Autodesk Fusion 360 part; units mm, degrees
(part 2 of 6)
  line L802 (34.113611, 287.460972) -> (34.113611, 286.790694)
  line L803 (27.199167, 285.555972) -> (27.128611, 285.59125)
  line L804 (18.485556, 226.85375) -> (18.626667, 226.783194)
  line L805 (12.311944, 223.114305) -> (12.206111, 223.149583)
  line L806 (40.675278, 262.907639) -> (40.675278, 263.260417)
  line L807 (41.557222, 261.672917) -> (41.310278, 261.708194)
  line L808 (41.310278, 261.708194) -> (41.169167, 261.814028)
  line L809 (25.011944, 250.454583) -> (25.047222, 250.384028)
  line L810 (35.277778, 273.490972) -> (34.713333, 275.325417)
  line L811 (34.713333, 275.325417) -> (34.148889, 273.490972)
  line L812 (34.148889, 273.490972) -> (35.277778, 273.490972)
  line L813 (31.75, 237.119583) -> (31.361944, 236.660972)
  line L814 (34.219444, 289.542361) -> (34.466389, 289.330694)
  line L815 (34.466389, 289.330694) -> (34.572222, 289.189583)
  line L816 (38.205833, 240.682639) -> (38.170556, 240.576805)
  line L817 (40.075556, 240.788472) -> (38.488056, 240.788472)
  line L818 (34.29, 287.990139) -> (34.395833, 287.990139)
  line L819 (39.123056, 244.457361) -> (39.017222, 244.457361)
  line L820 (25.964444, 250.419305) -> (25.999722, 250.384028)
  line L821 (25.964444, 253.312083) -> (25.964444, 250.595694)
  line L822 (32.243889, 286.190972) -> (32.490833, 285.90875)
  line L823 (32.490833, 285.90875) -> (32.808333, 285.697083)
  line L824 (24.659167, 285.59125) -> (24.553333, 285.626528)
  line L825 (31.361944, 231.969028) -> (31.4325, 231.93375)
  line L826 (41.310278, 264.777361) -> (41.557222, 264.847917)
  line L827 (41.169167, 261.814028) -> (40.922222, 262.166805)
  line L828 (40.922222, 262.166805) -> (40.781111, 262.590139)
  line L829 (38.770278, 244.210417) -> (38.735, 243.928194)
  line L830 (39.017222, 244.457361) -> (38.911389, 244.386805)
  line L831 (39.0525, 250.877917) -> (38.558611, 251.93625)
  line L832 (39.899167, 243.857639) -> (39.828611, 243.892917)
  line L833 (39.299444, 251.512917) -> (40.040278, 253.100417)
  line L834 (39.405278, 241.599861) -> (39.546389, 241.635139)
  line L835 (24.482778, 285.697083) -> (24.482778, 285.802917)
  line L836 (20.778611, 243.010972) -> (20.990278, 243.575417)
  line L837 (40.287222, 236.237639) -> (40.3225, 236.308194)
  line L838 (40.3225, 236.308194) -> (40.357778, 236.414028)
  line L839 (26.846389, 234.79125) -> (27.481389, 234.826528)
  line L840 (27.481389, 234.826528) -> (28.081111, 234.932361)
  line L841 (38.346944, 249.431528) -> (38.241111, 249.466805)
  line L842 (27.657778, 295.292639) -> (27.481389, 295.292639)
  line L843 (39.581667, 243.293194) -> (39.087778, 243.434305)
  line L844 (32.808333, 285.697083) -> (33.090556, 285.59125)
  line L845 (39.758056, 234.755972) -> (39.863889, 234.79125)
  line L846 (39.863889, 234.79125) -> (39.899167, 234.826528)
  line L847 (39.899167, 234.826528) -> (39.934444, 234.897083)
  line L848 (39.299444, 250.736805) -> (39.37, 250.772083)
  line L849 (39.37, 250.772083) -> (39.440556, 250.807361)
  line L850 (39.440556, 250.807361) -> (39.511111, 250.913194)
  line L851 (27.6225, 291.059305) -> (27.728333, 291.094583)
  line L852 (27.728333, 291.094583) -> (27.763611, 291.165139)
  line L853 (27.763611, 291.165139) -> (27.798889, 291.200417)
  line L854 (27.305, 291.200417) -> (27.340278, 291.129861)
  line L855 (39.934444, 234.897083) -> (39.934444, 235.002917)
  line L856 (38.664444, 234.755972) -> (39.652222, 234.755972)
  line L857 (22.577778, 229.252639) -> (22.507222, 229.429028)
  line L858 (22.507222, 229.429028) -> (22.507222, 229.605417)
  line L859 (34.113611, 238.107361) -> (34.360556, 238.742361)
  line L860 (28.081111, 247.385417) -> (27.481389, 247.455972)
  line L861 (27.481389, 247.455972) -> (26.846389, 247.49125)
  line L862 (40.005, 249.71375) -> (40.005, 249.607917)
  line L863 (40.005, 249.607917) -> (40.040278, 249.537361)
  line L864 (40.005, 251.93625) -> (40.005, 249.71375)
  line L865 (27.340278, 291.129861) -> (27.410833, 291.094583)
  line L866 (39.511111, 250.913194) -> (40.005, 251.93625)
  line L867 (29.845, 225.26625) -> (29.845, 223.643472)
  line L868 (16.051389, 286.825972) -> (16.051389, 286.296805)
  line L869 (27.516667, 228.723472) -> (27.410833, 228.723472)
  line L870 (20.990278, 243.575417) -> (21.2725, 244.139861)
  line L871 (39.0525, 226.85375) -> (38.170556, 226.85375)
  line L872 (34.113611, 293.634583) -> (34.007778, 293.52875)
  line L873 (28.716111, 247.244305) -> (29.280556, 247.032639)
  line L874 (20.990278, 238.707083) -> (20.778611, 239.306805)
  line L875 (41.874722, 261.77875) -> (41.945278, 261.884583)
  line L876 (34.713333, 241.494028) -> (34.713333, 240.788472)
  line L877 (34.713333, 240.788472) -> (34.678056, 240.118194)
  line L878 (34.678056, 240.118194) -> (34.536944, 239.412639)
  line L879 (34.536944, 239.412639) -> (34.360556, 238.742361)
  line L880 (34.360556, 238.742361) -> (34.113611, 238.107361)
  line L881 (34.113611, 238.107361) -> (33.831389, 237.472361)
  line L882 (33.831389, 237.472361) -> (33.478611, 236.872639)
  line L883 (33.478611, 236.872639) -> (33.055278, 236.308194)
  line L884 (33.055278, 236.308194) -> (32.596667, 235.779028)
  line L885 (32.596667, 235.779028) -> (32.102778, 235.285139)
  line L886 (32.102778, 235.285139) -> (31.573611, 234.861805)
  line L887 (31.573611, 234.861805) -> (31.009167, 234.438472)
  line L888 (31.009167, 234.438472) -> (30.374167, 234.120972)
  line L889 (30.374167, 234.120972) -> (29.739167, 233.83875)
  line L890 (29.739167, 233.83875) -> (29.104167, 233.591805)
  line L891 (29.104167, 233.591805) -> (28.398611, 233.450694)
  line L892 (28.398611, 233.450694) -> (27.728333, 233.344861)
  line L893 (27.728333, 233.344861) -> (27.022778, 233.274305)
  line L894 (27.022778, 233.274305) -> (26.317222, 233.309583)
  line L895 (26.317222, 233.309583) -> (25.646944, 233.380139)
  line L896 (25.646944, 233.380139) -> (24.976667, 233.52125)
  line L897 (24.976667, 233.52125) -> (24.306389, 233.697639)
  line L898 (24.306389, 233.697639) -> (23.636111, 233.979861)
  line L899 (23.636111, 233.979861) -> (23.036389, 234.262083)
  line L900 (23.036389, 234.262083) -> (22.436667, 234.650139)
  line L901 (22.436667, 234.650139) -> (21.872222, 235.073472)
  line L902 (21.872222, 235.073472) -> (21.343056, 235.532083)
  line L903 (21.343056, 235.532083) -> (20.884444, 236.025972)
  line L904 (20.884444, 236.025972) -> (20.461111, 236.590417)
  line L905 (20.461111, 236.590417) -> (20.073056, 237.154861)
  line L906 (20.073056, 237.154861) -> (19.755556, 237.789861)
  line L907 (19.755556, 237.789861) -> (19.473333, 238.424861)
  line L908 (19.473333, 238.424861) -> (19.261667, 239.095139)
  line L909 (19.261667, 239.095139) -> (19.120556, 239.765417)
  line L910 (19.120556, 239.765417) -> (19.014722, 240.470972)
  line L911 (19.014722, 240.470972) -> (18.979444, 241.14125)
  line L912 (18.979444, 241.14125) -> (19.014722, 241.846805)
  line L913 (19.014722, 241.846805) -> (19.120556, 242.552361)
  line L914 (19.120556, 242.552361) -> (19.261667, 243.222639)
  line L915 (19.261667, 243.222639) -> (19.473333, 243.892917)
  line L916 (19.473333, 243.892917) -> (19.755556, 244.527917)
  line L917 (19.755556, 244.527917) -> (20.073056, 245.127639)
  line L918 (20.073056, 245.127639) -> (20.461111, 245.727361)
  line L919 (20.461111, 245.727361) -> (20.884444, 246.291805)
  line L920 (20.884444, 246.291805) -> (21.343056, 246.785694)
  line L921 (21.343056, 246.785694) -> (21.872222, 247.244305)
  line L922 (21.872222, 247.244305) -> (22.436667, 247.667639)
  line L923 (22.436667, 247.667639) -> (23.036389, 248.020417)
  line L924 (23.036389, 248.020417) -> (23.636111, 248.337917)
  line L925 (23.636111, 248.337917) -> (24.306389, 248.584861)
  line L926 (24.306389, 248.584861) -> (24.976667, 248.796528)
  line L927 (24.976667, 248.796528) -> (25.646944, 248.937639)
  line L928 (25.646944, 248.937639) -> (26.317222, 249.008194)
  line L929 (26.317222, 249.008194) -> (27.022778, 249.043472)
  line L930 (27.022778, 249.043472) -> (27.728333, 248.972917)
  line L931 (27.728333, 248.972917) -> (28.398611, 248.867083)
  line L932 (28.398611, 248.867083) -> (29.104167, 248.690694)
  line L933 (29.104167, 248.690694) -> (29.739167, 248.479028)
  line L934 (29.739167, 248.479028) -> (30.374167, 248.196805)
  line L935 (30.374167, 248.196805) -> (31.009167, 247.844028)
  line L936 (31.009167, 247.844028) -> (31.573611, 247.455972)
  line L937 (31.573611, 247.455972) -> (32.102778, 247.032639)
  line L938 (32.102778, 247.032639) -> (32.596667, 246.53875)
  line L939 (32.596667, 246.53875) -> (33.055278, 246.009583)
  line L940 (33.055278, 246.009583) -> (33.478611, 245.445139)
  line L941 (33.478611, 245.445139) -> (33.831389, 244.845417)
  line L942 (33.831389, 244.845417) -> (34.113611, 244.210417)
  line L943 (34.113611, 244.210417) -> (34.360556, 243.540139)
  line L944 (34.360556, 243.540139) -> (34.536944, 242.869861)
  line L945 (34.536944, 242.869861) -> (34.678056, 242.199583)
  line L946 (34.678056, 242.199583) -> (34.713333, 241.494028)
  line L947 (1.446389, 282.945417) -> (14.322778, 295.821805)
  line L948 (39.828611, 243.963472) -> (39.793333, 244.034028)
  line L949 (15.980833, 223.643472) -> (16.086667, 223.537639)
  line L950 (39.934444, 243.822361) -> (39.899167, 243.857639)
  line L951 (39.087778, 243.434305) -> (39.581667, 243.293194)
  line L952 (33.161111, 240.541528) -> (33.090556, 239.906528)
  line L953 (39.793333, 244.034028) -> (39.6875, 244.31625)
  line L954 (29.280556, 247.032639) -> (28.716111, 247.244305)
  line L955 (28.716111, 247.244305) -> (28.081111, 247.385417)
  line L956 (40.216667, 243.892917) -> (40.146111, 243.822361)
  line L957 (39.0525, 265.624028) -> (39.123056, 265.694583)
  line L958 (33.408056, 289.824583) -> (32.949444, 289.71875)
  line L959 (32.949444, 289.71875) -> (32.596667, 289.542361)
  line L960 (20.672778, 295.821805) -> (19.261667, 295.821805)
  line L961 (13.899444, 289.048472) -> (6.596944, 281.745972)
  line L962 (43.285833, 281.745972) -> (43.991389, 282.486805)
  line L963 (25.153056, 229.675972) -> (25.576389, 231.087083)
  line L964 (40.251944, 243.963472) -> (40.216667, 243.892917)
  line L965 (15.5575, 225.372083) -> (15.522222, 225.336805)
  line L966 (27.446111, 285.732361) -> (27.410833, 285.661805)
  line L967 (23.459722, 289.824583) -> (21.2725, 289.824583)
  line L968 (37.076944, 261.602361) -> (37.076944, 261.567083)
  line L969 (27.163889, 289.471805) -> (27.093333, 289.365972)
  line L970 (30.1625, 295.11625) -> (30.091944, 295.186805)
  line L971 (30.091944, 295.186805) -> (30.021389, 295.257361)
  line L972 (30.021389, 295.257361) -> (29.809722, 295.292639)
  line L973 (26.387778, 252.077361) -> (26.387778, 253.20625)
  line L974 (23.918333, 251.265972) -> (24.341667, 252.677083)
  line L975 (24.765, 251.265972) -> (23.918333, 251.265972)
  line L976 (39.123056, 241.599861) -> (39.405278, 241.599861)
  line L977 (29.986111, 231.61625) -> (31.220833, 231.61625)
  line L978 (29.986111, 230.769583) -> (29.986111, 231.61625)
  line L979 (30.868056, 230.769583) -> (29.986111, 230.769583)
  line L980 (5.185833, 281.745972) -> (1.446389, 281.745972)
  line L981 (24.765, 289.648194) -> (24.729722, 289.577639)
  line L982 (25.294167, 289.612917) -> (25.153056, 289.754028)
  line L983 (36.5125, 226.959583) -> (36.477222, 227.030139)
  line L984 (37.853056, 289.71875) -> (37.958889, 289.789305)
  line L985 (30.338889, 250.525139) -> (30.338889, 253.382639)
  line L986 (30.127222, 250.313472) -> (30.233056, 250.313472)
  line L987 (27.305, 285.59125) -> (27.199167, 285.555972)
  line L988 (13.229167, 223.467083) -> (13.229167, 227.030139)
  line L989 (8.643056, 235.532083) -> (8.325556, 235.355694)
  line L990 (8.325556, 235.355694) -> (8.043333, 235.144028)
  line L991 (39.123056, 241.14125) -> (39.405278, 241.14125)
  line L992 (38.205833, 242.164305) -> (38.276389, 241.740972)
  line L993 (21.237222, 226.500972) -> (21.060833, 226.254028)
  line L994 (43.991389, 295.186805) -> (43.991389, 295.821805)
  line L995 (43.991389, 295.821805) -> (39.722778, 295.821805)
  line L996 (22.189722, 229.852361) -> (22.295556, 229.852361)
  line L997 (22.295556, 229.852361) -> (22.366111, 229.852361)
  line L998 (22.366111, 229.852361) -> (22.436667, 229.817083)
  line L999 (16.792222, 223.325972) -> (16.8275, 223.220139)
  line L1000 (16.8275, 223.220139) -> (16.898056, 223.149583)
  line L1001 (15.769167, 226.85375) -> (13.758333, 226.85375)
  line L1002 (38.311667, 228.794028) -> (38.4175, 228.75875)
  line L1003 (39.546389, 241.635139) -> (39.6875, 241.705694)
  line L1004 (15.804444, 227.382917) -> (13.581944, 227.382917)
  line L1005 (19.579167, 226.148194) -> (19.508611, 226.500972)
  line L1006 (19.508611, 226.500972) -> (19.332222, 226.85375)
  line L1007 (34.043056, 294.587083) -> (34.184167, 294.410694)
  line L1008 (9.913056, 223.467083) -> (9.913056, 223.36125)
  line L1009 (37.747222, 293.422917) -> (37.747222, 293.52875)
  line L1010 (37.747222, 293.52875) -> (37.711944, 293.599305)
  line L1011 (37.711944, 293.599305) -> (37.641389, 293.669861)
  line L1012 (16.051389, 226.924305) -> (16.086667, 226.994861)
  line L1013 (16.086667, 226.994861) -> (16.121944, 227.100694)
  line L1014 (22.154444, 229.217361) -> (22.083889, 229.570139)
  line L1015 (22.083889, 229.570139) -> (22.119167, 229.746528)
  line L1016 (22.119167, 229.746528) -> (22.189722, 229.852361)
  line L1017 (25.646944, 287.884305) -> (24.800278, 289.365972)
  line L1018 (27.763611, 291.165139) -> (27.728333, 291.094583)
  line L1019 (11.253611, 234.755972) -> (11.43, 234.403194)
  line L1020 (11.43, 234.403194) -> (11.535833, 234.085694)
  line L1021 (32.526111, 291.376805) -> (32.526111, 292.823194)
  line L1022 (13.335, 279.735139) -> (13.476111, 280.017361)
  line L1023 (39.6875, 244.31625) -> (39.793333, 244.034028)
  line L1024 (35.489444, 295.186805) -> (35.454167, 295.080972)
  line L1025 (35.665833, 226.889028) -> (35.418889, 226.85375)
  line L1026 (35.418889, 226.85375) -> (34.572222, 226.85375)
  line L1027 (29.950833, 294.79875) -> (29.809722, 294.763472)
  line L1028 (39.793333, 244.845417) -> (40.005, 244.669028)
  line L1029 (30.1625, 295.045694) -> (30.1625, 295.11625)
  line L1030 (39.934444, 243.822361) -> (40.040278, 243.787083)
  line L1031 (11.288889, 224.807639) -> (11.183056, 224.666528)
  line L1032 (3.104444, 222.549861) -> (1.446389, 220.891806)
  line L1033 (1.446389, 220.891806) -> (1.446389, 222.549861)
  line L1034 (1.446389, 222.549861) -> (3.104444, 222.549861)
  line L1035 (43.991389, 218.034306) -> (43.991389, 218.986806)
  line L1036 (8.043333, 235.144028) -> (7.796389, 234.897083)
  line L1037 (7.796389, 234.897083) -> (7.584722, 234.579583)
  line L1038 (7.584722, 234.579583) -> (7.443611, 234.262083)
  line L1039 (17.180278, 227.382917) -> (17.003889, 227.347639)
  line L1040 (17.003889, 227.347639) -> (16.862778, 227.277083)
  line L1041 (27.481389, 295.292639) -> (27.340278, 295.186805)
  line L1042 (27.340278, 295.186805) -> (27.305, 295.080972)
  line L1043 (27.305, 295.080972) -> (27.269722, 294.939861)
  line L1044 (29.809722, 295.292639) -> (27.657778, 295.292639)
  line L1045 (13.335, 257.898194) -> (13.229167, 258.180417)
  line L1046 (28.222222, 289.754028) -> (28.186944, 289.71875)
  line L1047 (28.398611, 248.867083) -> (27.728333, 248.972917)
  line L1048 (27.728333, 248.972917) -> (27.022778, 249.043472)
  line L1049 (27.022778, 249.043472) -> (26.317222, 249.008194)
  line L1050 (26.317222, 249.008194) -> (25.646944, 248.937639)
  line L1051 (36.5125, 227.277083) -> (36.477222, 227.241805)
  line L1052 (36.477222, 227.241805) -> (36.477222, 227.135972)
  line L1053 (39.0525, 227.382917) -> (36.83, 227.382917)
  line L1054 (34.219444, 292.999583) -> (34.572222, 293.352361)
  line L1055 (11.535833, 234.085694) -> (11.606389, 233.732917)
  line L1056 (8.748889, 223.396528) -> (8.748889, 223.255417)
  line L1057 (38.735, 244.810139) -> (39.087778, 244.915972)
  line L1058 (27.022778, 253.170972) -> (27.128611, 253.135694)
  line L1059 (8.043333, 235.144028) -> (8.325556, 235.355694)
  line L1060 (8.325556, 235.355694) -> (8.643056, 235.532083)
  line L1061 (35.595278, 272.432639) -> (35.630556, 272.362083)
  line L1062 (35.630556, 272.362083) -> (35.701111, 272.291528)
  line L1063 (39.087778, 244.915972) -> (39.405278, 244.95125)
  line L1064 (34.6075, 289.08375) -> (34.572222, 289.189583)
  line L1065 (34.572222, 289.189583) -> (34.466389, 289.330694)
  line L1066 (34.078333, 285.732361) -> (34.29, 285.90875)
  line L1067 (34.29, 285.90875) -> (34.466389, 286.085139)
  line L1068 (31.220833, 229.111528) -> (29.986111, 229.111528)
  line L1069 (31.467778, 228.899861) -> (31.467778, 228.970417)
  line L1070 (31.467778, 228.970417) -> (31.4325, 229.040972)
  line L1071 (38.523333, 253.135694) -> (38.452778, 253.170972)
  line L1072 (38.452778, 253.170972) -> (38.4175, 253.20625)
  line L1073 (38.4175, 253.20625) -> (38.346944, 253.20625)
  line L1074 (25.964444, 288.44875) -> (26.67, 289.648194)
  line L1075 (27.6225, 231.61625) -> (27.6225, 230.769583)
  line L1076 (37.288611, 261.14375) -> (37.359167, 261.14375)
  line L1077 (7.443611, 234.262083) -> (7.337778, 233.909305)
  line L1078 (7.337778, 233.909305) -> (7.3025, 233.52125)
  line L1079 (36.935833, 281.745972) -> (31.996944, 281.745972)
  line L1080 (12.453056, 223.149583) -> (12.311944, 223.114305)
  line L1081 (19.085278, 223.290694) -> (19.191111, 223.184861)
  line L1082 (19.191111, 223.184861) -> (19.296944, 223.149583)
  line L1083 (40.146111, 243.822361) -> (40.216667, 243.892917)
  line L1084 (16.862778, 227.277083) -> (16.792222, 227.135972)
  line L1085 (15.5575, 225.58375) -> (15.5575, 225.513194)
  line L1086 (30.374167, 248.196805) -> (29.739167, 248.479028)
  line L1087 (29.739167, 248.479028) -> (29.104167, 248.690694)
  line L1088 (29.104167, 248.690694) -> (28.398611, 248.867083)
  line L1089 (27.375556, 286.014583) -> (26.281944, 287.884305)
  line L1090 (27.446111, 285.802917) -> (27.446111, 285.944028)
  line L1091 (27.375556, 284.885694) -> (24.235833, 281.745972)
  line L1092 (13.440833, 223.114305) -> (13.581944, 223.114305)
  line L1093 (13.229167, 227.030139) -> (13.229167, 223.467083)
  line L1094 (13.581944, 227.382917) -> (13.440833, 227.347639)
  line L1095 (38.488056, 249.502083) -> (38.4175, 249.466805)
  line L1096 (15.804444, 223.643472) -> (15.875, 223.643472)
  line L1097 (22.824722, 236.237639) -> (22.366111, 236.660972)
  line L1098 (40.357778, 242.234861) -> (40.287222, 242.622917)
  line L1099 (40.287222, 242.622917) -> (40.110833, 242.975694)
  line L1100 (40.110833, 242.975694) -> (39.899167, 243.187361)
  line L1101 (39.899167, 243.187361) -> (39.581667, 243.293194)
  line L1102 (34.642778, 265.200694) -> (33.584444, 261.567083)
  line L1103 (34.925, 265.377083) -> (34.819167, 265.377083)
  line L1104 (38.523333, 242.481805) -> (38.593889, 242.41125)
  line L1105 (23.530278, 229.358472) -> (23.389167, 229.182083)
  line L1106 (23.424444, 230.064028) -> (23.530278, 229.852361)
  line L1107 (33.584444, 272.25625) -> (33.690278, 272.25625)
  line L1108 (33.690278, 272.25625) -> (33.760833, 272.291528)
  line L1109 (21.872222, 235.073472) -> (22.436667, 234.650139)
  line L1110 (22.436667, 234.650139) -> (23.036389, 234.262083)
  line L1111 (23.036389, 234.262083) -> (23.636111, 233.979861)
  line L1112 (1.446389, 219.445417) -> (4.550833, 222.549861)
  line L1113 (4.550833, 222.549861) -> (9.454444, 222.549861)
  line L1114 (36.583056, 226.889028) -> (36.5125, 226.959583)
  line L1115 (38.523333, 249.537361) -> (38.558611, 249.749028)
  line L1116 (38.1, 249.749028) -> (38.135278, 249.537361)
  line L1117 (38.135278, 249.537361) -> (38.170556, 249.502083)
  line L1118 (38.170556, 249.502083) -> (38.241111, 249.466805)
  line L1119 (31.996944, 291.412083) -> (31.996944, 291.30625)
  line L1120 (34.007778, 272.961805) -> (35.418889, 272.961805)
  line L1121 (33.831389, 272.397361) -> (34.007778, 272.961805)
  line L1122 (33.655, 293.352361) -> (33.443333, 293.352361)
  line L1123 (25.999722, 250.384028) -> (26.070278, 250.313472)
  line L1124 (26.070278, 250.313472) -> (26.176111, 250.313472)
  line L1125 (15.522222, 225.336805) -> (15.451667, 225.301528)
  line L1126 (38.346944, 253.20625) -> (38.4175, 253.20625)
  line L1127 (38.276389, 240.753194) -> (38.488056, 240.788472)
  line L1128 (39.017222, 237.190139) -> (39.017222, 237.33125)
  line L1129 (27.798889, 291.200417) -> (27.763611, 291.165139)
  line L1130 (30.338889, 253.382639) -> (30.303611, 253.488472)
  line L1131 (30.303611, 253.488472) -> (30.268333, 253.559028)
  line L1132 (37.359167, 261.14375) -> (37.429722, 261.179028)
  line L1133 (37.429722, 261.179028) -> (37.500278, 261.284861)
  line L1134 (27.128611, 252.147917) -> (27.022778, 252.112639)
  line L1135 (27.022778, 252.112639) -> (26.881667, 252.077361)
  line L1136 (26.881667, 252.077361) -> (26.387778, 252.077361)
  line L1137 (26.916944, 253.20625) -> (27.022778, 253.170972)
  line L1138 (30.303611, 250.454583) -> (30.338889, 250.525139)
  line L1139 (29.950833, 250.384028) -> (29.986111, 250.34875)
  line L1140 (39.0525, 230.310972) -> (39.899167, 228.864583)
  line L1141 (21.237222, 226.500972) -> (21.448889, 226.712639)
  line L1142 (21.448889, 226.712639) -> (21.695833, 226.818472)
  line L1143 (21.695833, 226.818472) -> (21.9075, 226.85375)
  line L1144 (28.469167, 253.594305) -> (28.539722, 253.594305)
  line L1145 (25.999722, 253.52375) -> (25.964444, 253.417917)
  line L1146 (25.964444, 253.417917) -> (25.964444, 253.312083)
  line L1147 (30.056667, 253.594305) -> (30.021389, 253.559028)
  line L1148 (30.021389, 253.559028) -> (29.950833, 253.488472)
  line L1149 (27.199167, 252.183194) -> (27.128611, 252.147917)
  line L1150 (20.496389, 241.14125) -> (20.531667, 241.77625)
  line L1151 (31.009167, 234.438472) -> (31.573611, 234.861805)
  line L1152 (31.573611, 234.861805) -> (32.102778, 235.285139)
  line L1153 (32.102778, 235.285139) -> (32.596667, 235.779028)
  line L1154 (31.361944, 245.656805) -> (31.75, 245.198194)
  line L1155 (27.798889, 291.376805) -> (27.798889, 291.30625)
  line L1156 (26.846389, 234.79125) -> (26.246667, 234.826528)
  line L1157 (33.655, 287.990139) -> (34.29, 287.990139)
  line L1158 (30.233056, 250.313472) -> (30.303611, 250.384028)
  line L1159 (30.303611, 250.384028) -> (30.303611, 250.454583)
  line L1160 (38.276389, 240.365139) -> (38.452778, 240.329861)
  line L1161 (38.488056, 240.788472) -> (38.276389, 240.753194)
  line L1162 (38.276389, 240.753194) -> (38.241111, 240.717917)
  line L1163 (38.241111, 240.717917) -> (38.205833, 240.682639)
  line L1164 (31.996944, 294.939861) -> (31.996944, 291.412083)
  line L1165 (32.385, 295.292639) -> (32.208611, 295.292639)
  line L1166 (16.051389, 286.296805) -> (11.535833, 281.745972)
  line L1167 (39.0525, 237.154861) -> (39.017222, 237.190139)
  line L1168 (39.616944, 244.915972) -> (39.440556, 244.95125)
  line L1169 (40.287222, 244.034028) -> (40.216667, 244.280972)
  line L1170 (40.216667, 244.280972) -> (40.146111, 244.457361)
  line L1171 (40.040278, 243.787083) -> (40.146111, 243.822361)
  line L1172 (22.789444, 229.111528) -> (22.718889, 229.146805)
  line L1173 (22.718889, 229.146805) -> (22.577778, 229.252639)
  line L1174 (34.6075, 286.367361) -> (34.642778, 286.614305)
  line L1175 (35.348333, 285.873472) -> (35.348333, 285.732361)
  line L1176 (35.348333, 285.732361) -> (35.418889, 285.626528)
  line L1177 (35.418889, 285.626528) -> (35.489444, 285.59125)
  line L1178 (16.792222, 227.135972) -> (16.792222, 226.994861)
  line L1179 (18.273889, 227.382917) -> (17.180278, 227.382917)
  line L1180 (21.343056, 235.532083) -> (21.872222, 235.073472)
  line L1181 (31.115, 230.628472) -> (31.079722, 230.699028)
  line L1182 (31.079722, 230.699028) -> (31.044444, 230.734305)
  line L1183 (31.044444, 230.734305) -> (30.868056, 230.769583)
  line L1184 (38.205833, 240.682639) -> (38.241111, 240.717917)
  line L1185 (32.138056, 237.613472) -> (32.455556, 238.177917)
  line L1186 (32.455556, 238.177917) -> (32.737778, 238.707083)
  line L1187 (4.974167, 218.034306) -> (1.446389, 218.034306)
  line L1188 (1.446389, 218.034306) -> (1.446389, 219.445417)
  line L1189 (39.722778, 295.821805) -> (39.334722, 295.43375)
  line L1190 (39.334722, 290.494861) -> (43.991389, 295.186805)
  line L1191 (27.587222, 223.749305) -> (27.834167, 223.925694)
  line L1192 (27.375556, 223.67875) -> (27.587222, 223.749305)
  line L1193 (21.448889, 287.707917) -> (21.448889, 286.085139)
  line L1194 (21.448889, 286.085139) -> (23.495, 286.085139)
  line L1195 (23.495, 286.085139) -> (23.565556, 286.085139)
  line L1196 (33.760833, 292.823194) -> (34.219444, 292.999583)
  line L1197 (12.135556, 223.184861) -> (12.065, 223.255417)
  line L1198 (37.923611, 222.549861) -> (41.204444, 222.549861)
  line L1199 (42.650833, 222.549861) -> (43.991389, 222.549861)
  line L1200 (43.991389, 222.549861) -> (43.991389, 281.745972)
  line L1201 (39.228889, 265.694583) -> (39.299444, 265.659305)
  line L1202 (29.986111, 250.34875) -> (30.021389, 250.313472)
  line L1203 (30.021389, 250.313472) -> (30.127222, 250.313472)
  line L1204 (34.854444, 222.549861) -> (30.374167, 218.034306)
  line L1205 (30.374167, 218.034306) -> (25.435278, 218.034306)
  line L1206 (25.435278, 218.034306) -> (29.950833, 222.549861)
  line L1207 (29.950833, 222.549861) -> (31.855833, 222.549861)
  line L1208 (33.760833, 272.291528) -> (33.796111, 272.326805)
  line L1209 (33.796111, 272.326805) -> (33.831389, 272.397361)
  line L1210 (33.302222, 272.467917) -> (33.3375, 272.362083)
  line L1211 (38.241111, 291.094583) -> (37.958889, 291.059305)
  line L1212 (35.348333, 289.577639) -> (35.348333, 289.507083)
  line L1213 (35.56, 289.824583) -> (35.489444, 289.789305)
  line L1214 (35.489444, 289.789305) -> (35.418889, 289.754028)
  line L1215 (20.6375, 239.906528) -> (20.778611, 239.306805)
  line L1216 (20.778611, 239.306805) -> (20.990278, 238.707083)
  line L1217 (29.315833, 285.732361) -> (29.315833, 285.838194)
  line L1218 (24.765, 289.648194) -> (24.800278, 289.71875)
  line L1219 (16.121944, 223.255417) -> (16.157222, 223.396528)
  line L1220 (13.581944, 223.114305) -> (15.769167, 223.114305)
  line L1221 (13.229167, 223.467083) -> (13.264444, 223.325972)
  line L1222 (39.0525, 265.624028) -> (38.981944, 265.553472)
  line L1223 (42.051111, 262.343194) -> (42.015833, 262.131528)
  line L1224 (17.885833, 224.913472) -> (19.085278, 223.290694)
  line L1225 (17.321389, 224.913472) -> (17.885833, 224.913472)
  line L1226 (17.321389, 223.467083) -> (17.321389, 224.913472)
  line L1227 (17.074444, 223.114305) -> (17.180278, 223.149583)
  line L1228 (29.845, 225.760139) -> (31.326667, 225.760139)
  line L1229 (24.800278, 289.71875) -> (24.906111, 289.789305)
  line L1230 (13.758333, 225.26625) -> (13.758333, 223.643472)
  line L1231 (31.397222, 228.75875) -> (31.4325, 228.75875)
  line L1232 (17.180278, 223.149583) -> (17.215556, 223.184861)
  line L1233 (17.215556, 223.184861) -> (17.286111, 223.220139)
  line L1234 (39.264167, 237.01375) -> (39.334722, 237.01375)
  line L1235 (39.334722, 237.01375) -> (39.405278, 237.049028)
  line L1236 (39.405278, 237.049028) -> (39.475833, 237.119583)
  line L1237 (39.475833, 237.119583) -> (39.511111, 237.295972)
  line L1238 (9.383889, 235.673194) -> (8.995833, 235.637917)
  line L1239 (8.995833, 235.637917) -> (8.643056, 235.532083)
  line L1240 (12.065, 223.255417) -> (12.065, 223.325972)
  line L1241 (22.507222, 223.960972) -> (22.577778, 224.137361)
  line L1242 (29.5275, 293.246528) -> (29.421667, 293.21125)
  line L1243 (34.360556, 288.695694) -> (34.501667, 288.730972)
  line L1244 (34.501667, 288.730972) -> (34.572222, 288.801528)
  line L1245 (28.2575, 253.347361) -> (28.292778, 253.488472)
  line L1246 (37.429722, 293.705139) -> (37.641389, 293.669861)
  line L1247 (31.4325, 228.75875) -> (31.467778, 228.829305)
  line L1248 (31.467778, 228.829305) -> (31.467778, 228.899861)
  line L1249 (29.845, 228.723472) -> (31.220833, 228.723472)
  line L1250 (38.523333, 236.660972) -> (40.075556, 236.660972)
  line L1251 (24.906111, 289.789305) -> (25.011944, 289.824583)
  line L1252 (12.065, 223.325972) -> (12.065, 223.431805)
  line L1253 (13.264444, 223.325972) -> (13.335, 223.184861)
  line L1254 (13.335, 223.184861) -> (13.440833, 223.114305)
  line L1255 (35.454167, 294.939861) -> (35.454167, 291.376805)
  line L1256 (32.243889, 258.497917) -> (32.208611, 258.180417)
  line L1257 (35.418889, 289.754028) -> (35.348333, 289.648194)
  line L1258 (37.958889, 294.763472) -> (38.1, 294.763472)
  line L1259 (38.1, 294.763472) -> (38.205833, 294.834028)
  line L1260 (11.43, 234.403194) -> (11.253611, 234.755972)
  line L1261 (11.253611, 234.755972) -> (11.006667, 235.038194)
  line L1262 (38.276389, 294.869305) -> (38.205833, 294.834028)
  line L1263 (29.598056, 228.970417) -> (29.598056, 228.864583)
  line L1264 (29.598056, 228.864583) -> (29.668611, 228.75875)
  line L1265 (29.668611, 228.75875) -> (29.739167, 228.723472)
  line L1266 (39.581667, 230.310972) -> (39.616944, 230.34625)
  line L1267 (40.216667, 229.182083) -> (39.581667, 230.310972)
  line L1268 (40.251944, 229.146805) -> (40.216667, 229.182083)
  line L1269 (40.3225, 228.970417) -> (40.3225, 229.040972)
  line L1270 (40.3225, 229.040972) -> (40.287222, 229.07625)
  line L1271 (30.021389, 295.257361) -> (30.091944, 295.186805)
  line L1272 (38.170556, 249.502083) -> (38.135278, 249.537361)
  line L1273 (27.269722, 291.376805) -> (27.269722, 294.939861)
  line L1274 (25.047222, 250.384028) -> (25.117778, 250.313472)
  line L1275 (21.59, 237.613472) -> (21.2725, 238.177917)
  line L1276 (32.243889, 279.135417) -> (32.243889, 258.497917)
  line L1277 (19.120556, 242.552361) -> (19.014722, 241.846805)
  line L1278 (19.014722, 241.846805) -> (18.979444, 241.14125)
  line L1279 (23.565556, 230.487361) -> (23.318611, 230.593194)
  line L1280 (23.142222, 228.723472) -> (23.530278, 228.794028)
  line L1281 (23.671389, 247.526528) -> (23.106944, 247.209028)
  line L1282 (23.106944, 247.209028) -> (22.577778, 246.820972)
  line L1283 (20.990278, 243.575417) -> (20.778611, 243.010972)
  line L1284 (20.778611, 243.010972) -> (20.6375, 242.375972)
  line L1285 (28.680833, 230.699028) -> (28.716111, 230.628472)
  line L1286 (38.382222, 236.625694) -> (38.523333, 236.660972)
  line L1287 (30.091944, 295.186805) -> (30.1625, 295.11625)
  line L1288 (40.428333, 249.537361) -> (40.463611, 249.607917)
  line L1289 (40.463611, 249.607917) -> (40.463611, 249.71375)
  line L1290 (40.463611, 249.71375) -> (40.463611, 252.959305)
  line L1291 (40.216667, 249.431528) -> (40.357778, 249.466805)
  line L1292 (40.357778, 249.466805) -> (40.428333, 249.537361)
  line L1293 (8.043333, 231.93375) -> (7.796389, 232.180694)
  line L1294 (27.481389, 295.292639) -> (27.657778, 295.292639)
  line L1295 (41.627778, 263.013472) -> (41.521944, 263.04875)
  line L1296 (40.287222, 229.07625) -> (40.251944, 229.146805)
  line L1297 (39.440556, 250.807361) -> (39.37, 250.772083)
  line L1298 (8.396111, 227.382917) -> (8.607778, 227.347639)
  line L1299 (8.607778, 227.347639) -> (8.678333, 227.277083)
  line L1300 (20.214167, 225.230972) -> (20.284722, 225.689583)
  line L1301 (20.284722, 225.689583) -> (20.390556, 226.148194)
  line L1302 (20.390556, 226.148194) -> (20.672778, 226.677361)
  line L1303 (38.664444, 242.305417) -> (38.593889, 242.41125)
  line L1304 (38.593889, 242.41125) -> (38.523333, 242.481805)
  line L1305 (38.523333, 242.481805) -> (38.452778, 242.481805)
  line L1306 (39.123056, 241.599861) -> (39.017222, 241.599861)
  line L1307 (37.747222, 293.52875) -> (37.747222, 293.422917)
  line L1308 (28.398611, 227.382917) -> (28.292778, 227.347639)
  line L1309 (27.199167, 231.722083) -> (27.199167, 228.970417)
  line L1310 (27.481389, 232.004305) -> (27.340278, 232.004305)
  line L1311 (27.340278, 232.004305) -> (27.234444, 231.93375)
  line L1312 (27.834167, 223.925694) -> (28.010556, 224.137361)
  line L1313 (40.040278, 245.480417) -> (40.075556, 245.409861)
  line L1314 (40.075556, 245.409861) -> (40.146111, 245.339305)
  line L1315 (40.146111, 245.339305) -> (40.216667, 245.304028)
  line L1316 (40.216667, 245.304028) -> (40.287222, 245.304028)
  line L1317 (40.3225, 253.20625) -> (40.251944, 253.20625)
  line L1318 (29.104167, 251.583472) -> (28.680833, 252.465417)
  line L1319 (27.163889, 223.643472) -> (27.375556, 223.67875)
  line L1320 (39.475833, 237.119583) -> (39.405278, 237.049028)
  line L1321 (22.895278, 228.688194) -> (22.613056, 228.75875)
  line L1322 (22.613056, 228.75875) -> (22.366111, 228.899861)
  line L1323 (22.366111, 228.899861) -> (22.154444, 229.217361)
  line L1324 (40.287222, 272.25625) -> (40.393056, 272.291528)
  line L1325 (40.393056, 272.291528) -> (40.428333, 272.326805)
  line L1326 (13.264444, 223.325972) -> (13.229167, 223.467083)
  line L1327 (33.866667, 289.154305) -> (34.113611, 288.872083)
  line L1328 (42.051111, 263.013472) -> (41.733611, 263.013472)
  line L1329 (35.56, 289.824583) -> (35.665833, 289.789305)
  line L1330 (23.918333, 229.993472) -> (23.777222, 230.310972)
  line L1331 (23.777222, 230.310972) -> (23.565556, 230.487361)
  line L1332 (25.964444, 287.390417) -> (25.011944, 285.767639)
  line L1333 (29.421667, 251.477639) -> (29.492222, 251.583472)
  line L1334 (29.104167, 251.583472) -> (29.139444, 251.512917)
  line L1335 (27.199167, 228.970417) -> (27.199167, 228.864583)
  line L1336 (27.199167, 228.864583) -> (27.269722, 228.75875)
  line L1337 (27.269722, 228.75875) -> (27.340278, 228.723472)
  line L1338 (32.102778, 236.37875) -> (32.526111, 236.872639)
  line L1339 (32.526111, 236.872639) -> (32.914167, 237.401805)
  line L1340 (38.840833, 243.010972) -> (38.981944, 242.975694)
  line L1341 (40.040278, 240.329861) -> (40.181389, 240.329861)
  line L1342 (31.150278, 246.820972) -> (30.585833, 247.209028)
  line L1343 (30.585833, 247.209028) -> (30.021389, 247.526528)
  line L1344 (28.363333, 250.313472) -> (28.328056, 250.34875)
  line L1345 (36.935833, 281.745972) -> (31.996944, 281.745972)
  line L1346 (30.585833, 281.745972) -> (25.646944, 281.745972)
  line L1347 (24.235833, 281.745972) -> (19.296944, 281.745972)
  line L1348 (28.363333, 250.313472) -> (28.469167, 250.313472)
  line L1349 (28.2575, 253.347361) -> (28.2575, 250.560417)
  line L1350 (38.1, 249.749028) -> (38.1, 252.924028)
  line L1351 (32.243889, 287.707917) -> (32.279167, 287.990139)
  line L1352 (32.279167, 287.990139) -> (32.349722, 288.272361)
  line L1353 (24.906111, 228.829305) -> (25.011944, 229.252639)
  line L1354 (24.694444, 228.723472) -> (24.765, 228.723472)
  line L1355 (18.415, 225.442639) -> (18.238611, 225.407361)
  line L1356 (29.633333, 231.93375) -> (29.598056, 231.827917)
  line L1357 (29.598056, 231.827917) -> (29.598056, 231.757361)
  line L1358 (31.220833, 232.004305) -> (29.845, 232.004305)
  line L1359 (33.478611, 238.60125) -> (33.690278, 239.200972)
  line L1360 (33.690278, 239.200972) -> (33.831389, 239.835972)
  line L1361 (35.983333, 294.763472) -> (37.958889, 294.763472)
  line L1362 (35.983333, 293.705139) -> (35.983333, 294.763472)
  line L1363 (37.429722, 293.705139) -> (35.983333, 293.705139)
  line L1364 (31.326667, 225.760139) -> (31.538333, 225.724861)
  line L1365 (12.946944, 281.745972) -> (16.086667, 284.885694)
  line L1366 (10.724444, 235.249861) -> (11.006667, 235.038194)
  line L1367 (11.006667, 235.038194) -> (11.253611, 234.755972)
  line L1368 (19.261667, 295.821805) -> (5.185833, 281.745972)
  line L1369 (34.043056, 294.587083) -> (34.184167, 294.410694)
  line L1370 (34.184167, 294.410694) -> (34.219444, 294.234305)
  line L1371 (39.264167, 276.665972) -> (39.193611, 276.736528)
  line L1372 (39.193611, 276.736528) -> (39.087778, 276.771805)
  line L1373 (28.645556, 227.206528) -> (28.680833, 227.135972)
  line L1374 (25.011944, 285.767639) -> (24.906111, 285.626528)
  line L1375 (13.264444, 227.17125) -> (13.299722, 227.277083)
  line L1376 (22.577778, 224.349028) -> (22.577778, 225.019305)
  line L1377 (35.736389, 285.59125) -> (35.665833, 285.555972)
  line L1378 (39.405278, 237.049028) -> (39.334722, 237.01375)
  line L1379 (31.996944, 281.745972) -> (35.136667, 284.885694)
  line L1380 (28.2575, 250.560417) -> (28.2575, 253.347361)
  line L1381 (28.680833, 252.465417) -> (28.680833, 250.560417)
  line L1382 (35.136667, 284.885694) -> (39.334722, 284.885694)
  line L1383 (39.899167, 242.234861) -> (39.863889, 242.446528)
  line L1384 (28.292778, 227.347639) -> (28.398611, 227.382917)
  line L1385 (23.353889, 232.004305) -> (23.495, 231.93375)
  line L1386 (23.495, 231.93375) -> (23.671389, 231.792639)
  line L1387 (23.671389, 231.792639) -> (23.8125, 231.61625)
  line L1388 (36.300833, 261.46125) -> (36.336111, 261.390694)
  line L1389 (36.336111, 261.390694) -> (36.300833, 261.284861)
  line L1390 (36.300833, 261.284861) -> (36.265556, 261.214305)
  line L1391 (36.265556, 261.214305) -> (36.159722, 261.14375)
  line L1392 (36.159722, 261.14375) -> (36.053889, 261.14375)
  line L1393 (36.053889, 261.14375) -> (35.983333, 261.14375)
  line L1394 (35.983333, 261.14375) -> (35.912778, 261.179028)
  line L1395 (35.912778, 261.179028) -> (35.842222, 261.249583)
  line L1396 (35.842222, 261.249583) -> (35.806944, 261.320139)
  line L1397 (35.806944, 261.320139) -> (35.630556, 261.849305)
  line L1398 (35.630556, 261.849305) -> (34.219444, 261.849305)
  line L1399 (34.219444, 261.849305) -> (34.043056, 261.284861)
  line L1400 (34.043056, 261.284861) -> (34.007778, 261.214305)
  line L1401 (34.007778, 261.214305) -> (33.9725, 261.179028)
  line L1402 (33.9725, 261.179028) -> (33.866667, 261.14375)
  line L1403 (33.866667, 261.14375) -> (33.796111, 261.14375)
  line L1404 (33.796111, 261.14375) -> (33.619722, 261.179028)
  line L1405 (33.619722, 261.179028) -> (33.549167, 261.249583)
  line L1406 (33.549167, 261.249583) -> (33.513889, 261.355417)
  line L1407 (33.513889, 261.355417) -> (33.549167, 261.46125)
  line L1408 (33.549167, 261.46125) -> (33.584444, 261.567083)
  line L1409 (33.584444, 261.567083) -> (34.642778, 265.200694)
  line L1410 (34.642778, 265.200694) -> (34.678056, 265.27125)
  line L1411 (34.678056, 265.27125) -> (34.748611, 265.341805)
  line L1412 (34.748611, 265.341805) -> (34.819167, 265.377083)
  line L1413 (34.819167, 265.377083) -> (34.925, 265.377083)
  line L1414 (34.925, 265.377083) -> (34.995556, 265.377083)
  line L1415 (34.995556, 265.377083) -> (35.066111, 265.341805)
  line L1416 (35.066111, 265.341805) -> (35.136667, 265.235972)
  line L1417 (35.136667, 265.235972) -> (35.171944, 265.130139)
  line L1418 (35.171944, 265.130139) -> (36.300833, 261.531805)
  line L1419 (36.300833, 261.531805) -> (36.300833, 261.46125)
  line L1420 (22.754167, 225.548472) -> (22.895278, 225.548472)
  line L1421 (33.3375, 287.566805) -> (33.408056, 287.49625)
  line L1422 (33.443333, 287.954861) -> (33.372778, 287.919583)
  line L1423 (29.174722, 251.442361) -> (29.139444, 251.512917)
  line L1424 (39.264167, 226.889028) -> (39.0525, 226.85375)
  line L1425 (29.386389, 293.705139) -> (29.492222, 293.634583)
  line L1426 (24.765, 251.265972) -> (23.918333, 251.265972)
  line L1427 (23.459722, 285.555972) -> (23.706667, 285.59125)
  line L1428 (23.706667, 285.59125) -> (23.777222, 285.626528)
  line L1429 (37.112222, 261.179028) -> (37.041667, 261.284861)
  line L1430 (20.6375, 242.375972) -> (20.531667, 241.77625)
  line L1431 (20.531667, 241.77625) -> (20.496389, 241.14125)
  line L1432 (29.139444, 251.512917) -> (29.104167, 251.583472)
  line L1433 (41.345556, 275.325417) -> (41.874722, 273.490972)
  line L1434 (27.093333, 289.754028) -> (26.9875, 289.789305)
  line L1435 (26.9875, 289.789305) -> (26.916944, 289.824583)
  line L1436 (29.351111, 293.175972) -> (29.21, 293.175972)
  line L1437 (23.353889, 230.134583) -> (23.212778, 230.169861)
  line L1438 (23.212778, 230.169861) -> (22.789444, 230.275694)
  line L1439 (22.789444, 230.275694) -> (22.648333, 230.34625)
  line L1440 (33.302222, 287.707917) -> (33.3375, 287.566805)
  line L1441 (21.695833, 223.67875) -> (21.942778, 223.643472)
  line L1442 (13.440833, 227.347639) -> (13.299722, 227.277083)
  line L1443 (30.868056, 230.381528) -> (29.986111, 230.381528)
  line L1444 (33.478611, 287.460972) -> (33.513889, 287.460972)
  line L1445 (33.513889, 287.460972) -> (33.655, 287.460972)
  line L1446 (25.011944, 289.824583) -> (24.906111, 289.789305)
  line L1447 (24.765, 289.471805) -> (24.800278, 289.365972)
  line L1448 (24.906111, 289.789305) -> (24.800278, 289.71875)
  line L1449 (35.630556, 295.292639) -> (35.806944, 295.292639)
  line L1450 (32.878889, 227.241805) -> (32.914167, 227.277083)
  line L1451 (27.798889, 293.175972) -> (27.798889, 291.376805)
  line L1452 (28.398611, 227.382917) -> (28.539722, 227.347639)
  line L1453 (30.726944, 289.824583) -> (30.938611, 289.754028)
  line L1454 (42.368611, 264.918472) -> (42.192222, 265.130139)
  line L1455 (28.680833, 250.560417) -> (28.680833, 252.465417)
  line L1456 (28.469167, 250.313472) -> (28.539722, 250.313472)
  line L1457 (35.524722, 291.094583) -> (35.454167, 291.235694)
  line L1458 (25.011944, 235.073472) -> (24.412222, 235.285139)
  line L1459 (43.991389, 287.390417) -> (38.346944, 281.745972)
  line L1460 (43.991389, 281.745972) -> (43.991389, 282.486805)
  line L1461 (37.076944, 261.602361) -> (38.981944, 265.553472)
  line L1462 (35.771667, 227.030139) -> (35.771667, 226.994861)
  line L1463 (35.771667, 226.994861) -> (35.736389, 226.924305)
  line L1464 (39.334722, 237.01375) -> (39.264167, 237.01375)
  line L1465 (33.478611, 245.445139) -> (33.055278, 246.009583)
  line L1466 (24.482778, 285.90875) -> (24.553333, 286.049861)
  line L1467 (39.334722, 290.494861) -> (43.991389, 295.186805)
  line L1468 (38.488056, 241.388194) -> (38.276389, 241.740972)
  line L1469 (29.421667, 285.59125) -> (29.351111, 285.661805)
  line L1470 (28.645556, 230.734305) -> (28.680833, 230.699028)
  line L1471 (26.67, 289.648194) -> (25.964444, 288.44875)
  line L1472 (26.916944, 289.824583) -> (26.811111, 289.789305)
  line L1473 (29.245278, 251.442361) -> (29.280556, 251.442361)
  line L1474 (28.680833, 252.465417) -> (29.104167, 251.583472)
  line L1475 (40.181389, 236.202361) -> (40.040278, 236.167083)
  line L1476 (35.171944, 265.130139) -> (35.136667, 265.235972)
  line L1477 (19.014722, 226.324583) -> (19.05, 226.148194)
  line L1478 (39.334722, 289.08375) -> (39.334722, 290.494861)
  line L1479 (18.944167, 226.500972) -> (19.014722, 226.324583)
  line L1480 (38.170556, 285.59125) -> (38.064722, 285.555972)
  line L1481 (15.910278, 226.85375) -> (15.769167, 226.85375)
  line L1482 (35.454167, 294.939861) -> (35.454167, 295.080972)
  line L1483 (23.8125, 285.838194) -> (23.8125, 285.90875)
  line L1484 (23.8125, 285.90875) -> (23.777222, 285.979305)
  line L1485 (37.747222, 293.422917) -> (37.747222, 293.317083)
  line L1486 (37.429722, 261.179028) -> (37.359167, 261.14375)
  line L1487 (31.361944, 236.660972) -> (31.75, 237.119583)
  line L1488 (31.75, 237.119583) -> (32.138056, 237.613472)
  line L1489 (23.530278, 228.794028) -> (23.8125, 229.040972)
  line L1490 (23.8125, 229.040972) -> (23.953611, 229.323194)
  line L1491 (29.562778, 285.555972) -> (29.421667, 285.59125)
  line L1492 (39.863889, 235.179305) -> (39.899167, 235.144028)
  line L1493 (29.351111, 285.661805) -> (29.315833, 285.732361)
  line L1494 (21.9075, 226.85375) -> (21.695833, 226.818472)
  line L1495 (38.4175, 249.466805) -> (38.346944, 249.431528)
  line L1496 (30.091944, 294.834028) -> (30.1625, 294.939861)
  line L1497 (30.1625, 294.939861) -> (30.1625, 295.045694)
  line L1498 (27.798889, 294.763472) -> (29.809722, 294.763472)
  line L1499 (27.798889, 293.705139) -> (27.798889, 294.763472)
  line L1500 (38.311667, 291.165139) -> (38.276389, 291.129861)
  line L1501 (28.469167, 230.769583) -> (28.645556, 230.734305)
  line L1502 (42.051111, 262.343194) -> (42.051111, 263.013472)
  line L1503 (39.899167, 235.144028) -> (39.934444, 235.073472)
  line L1504 (39.6875, 235.214583) -> (39.863889, 235.179305)
  line L1505 (22.86, 226.254028) -> (22.965833, 226.289305)
  line L1506 (22.965833, 226.289305) -> (23.071667, 226.359861)
  line L1507 (23.071667, 226.359861) -> (23.106944, 226.465694)
  line L1508 (22.154444, 226.818472) -> (21.9075, 226.85375)
  line L1509 (38.205833, 295.257361) -> (38.276389, 295.186805)
  line L1510 (23.636111, 286.085139) -> (23.565556, 286.085139)
  line L1511 (23.565556, 286.085139) -> (23.495, 286.085139)
  line L1512 (38.276389, 295.186805) -> (38.311667, 295.11625)
  line L1513 (38.664444, 235.214583) -> (39.6875, 235.214583)
  line L1514 (21.9075, 227.382917) -> (22.154444, 227.347639)
  line L1515 (22.154444, 227.347639) -> (22.401389, 227.277083)
  line L1516 (22.401389, 227.277083) -> (22.683611, 227.100694)
  line L1517 (38.664444, 236.167083) -> (38.664444, 235.214583)
  line L1518 (38.311667, 295.11625) -> (38.311667, 295.045694)
  line L1519 (29.845, 226.85375) -> (29.845, 225.760139)
  line L1520 (25.364722, 231.863194) -> (24.518056, 229.07625)
  line L1521 (25.576389, 232.004305) -> (25.505833, 232.004305)
  line L1522 (22.366111, 236.660972) -> (22.824722, 236.237639)
  line L1523 (22.824722, 236.237639) -> (23.318611, 235.884861)
  line L1524 (23.495, 286.085139) -> (21.448889, 286.085139)
  line L1525 (25.646944, 248.937639) -> (24.976667, 248.796528)
  line L1526 (24.976667, 248.796528) -> (24.306389, 248.584861)
  line L1527 (27.516667, 228.723472) -> (27.551944, 228.75875)
  line L1528 (27.551944, 228.75875) -> (27.587222, 228.794028)
  line L1529 (27.587222, 228.794028) -> (27.6225, 228.970417)
  line L1530 (38.311667, 295.045694) -> (38.311667, 294.904583)
  line L1531 (22.330833, 226.712639) -> (22.154444, 226.818472)
  line L1532 (37.817778, 285.873472) -> (37.817778, 287.707917)
  line L1533 (29.598056, 293.422917) -> (29.598056, 293.564028)
  line L1534 (29.598056, 293.564028) -> (29.5275, 293.599305)
  line L1535 (29.5275, 293.599305) -> (29.492222, 293.634583)
  line L1536 (29.492222, 293.634583) -> (29.386389, 293.705139)
  line L1537 (27.6225, 230.769583) -> (28.469167, 230.769583)
  line L1538 (39.863889, 234.79125) -> (39.758056, 234.755972)
  line L1539 (37.006389, 261.46125) -> (37.076944, 261.567083)
  line L1540 (31.996944, 226.85375) -> (31.855833, 226.85375)
  line L1541 (6.385278, 225.760139) -> (6.385278, 226.85375)
  line L1542 (7.831667, 225.760139) -> (6.385278, 225.760139)
  line L1543 (8.184444, 225.513194) -> (8.149167, 225.58375)
  line L1544 (19.579167, 223.396528) -> (19.579167, 223.325972)
  line L1545 (19.579167, 223.325972) -> (19.508611, 223.220139)
  line L1546 (19.508611, 223.220139) -> (19.438056, 223.184861)
  line L1547 (19.438056, 223.184861) -> (19.296944, 223.149583)
  line L1548 (19.296944, 223.149583) -> (19.191111, 223.184861)
  line L1549 (19.191111, 223.184861) -> (19.085278, 223.290694)
  line L1550 (19.085278, 223.290694) -> (17.885833, 224.913472)
  line L1551 (17.885833, 224.913472) -> (17.321389, 224.913472)
  line L1552 (17.321389, 224.913472) -> (17.321389, 223.467083)
  line L1553 (17.321389, 223.467083) -> (17.286111, 223.220139)
  line L1554 (17.286111, 223.220139) -> (17.215556, 223.184861)
  line L1555 (17.215556, 223.184861) -> (17.180278, 223.149583)
  line L1556 (17.180278, 223.149583) -> (17.074444, 223.114305)
  line L1557 (17.074444, 223.114305) -> (16.898056, 223.149583)
  line L1558 (16.898056, 223.149583) -> (16.8275, 223.220139)
  line L1559 (16.8275, 223.220139) -> (16.792222, 223.325972)
  line L1560 (16.792222, 223.325972) -> (16.792222, 223.396528)
  line L1561 (16.792222, 223.396528) -> (16.792222, 223.502361)
  line L1562 (16.792222, 223.502361) -> (16.792222, 226.994861)
  line L1563 (16.792222, 226.994861) -> (16.792222, 227.135972)
  line L1564 (16.792222, 227.135972) -> (16.862778, 227.277083)
  line L1565 (16.862778, 227.277083) -> (17.003889, 227.347639)
  line L1566 (17.003889, 227.347639) -> (17.180278, 227.382917)
  line L1567 (17.180278, 227.382917) -> (18.273889, 227.382917)
  line L1568 (18.273889, 227.382917) -> (18.697222, 227.312361)
  line L1569 (18.697222, 227.312361) -> (19.085278, 227.135972)
  line L1570 (19.085278, 227.135972) -> (19.332222, 226.85375)
  line L1571 (19.332222, 226.85375) -> (19.508611, 226.500972)
  line L1572 (19.508611, 226.500972) -> (19.579167, 226.148194)
  line L1573 (19.579167, 226.148194) -> (19.508611, 225.760139)
  line L1574 (19.508611, 225.760139) -> (19.332222, 225.407361)
  line L1575 (19.332222, 225.407361) -> (18.979444, 225.089861)
  line L1576 (18.979444, 225.089861) -> (18.520833, 224.913472)
  line L1577 (18.520833, 224.913472) -> (19.473333, 223.608194)
  line L1578 (19.473333, 223.608194) -> (19.508611, 223.572917)
  line L1579 (19.508611, 223.572917) -> (19.543889, 223.502361)
  line L1580 (19.543889, 223.502361) -> (19.579167, 223.396528)
  line L1581 (23.565556, 286.085139) -> (23.636111, 286.085139)
  line L1582 (23.636111, 286.085139) -> (23.777222, 285.979305)
  line L1583 (23.777222, 285.979305) -> (23.8125, 285.90875)
  line L1584 (22.577778, 226.430417) -> (22.330833, 226.712639)
  line L1585 (13.193889, 258.497917) -> (13.193889, 279.135417)
  line L1586 (39.934444, 234.897083) -> (39.899167, 234.826528)
  line L1587 (35.665833, 291.059305) -> (35.524722, 291.094583)
  line L1588 (38.276389, 228.899861) -> (38.276389, 228.864583)
  line L1589 (38.276389, 228.864583) -> (38.311667, 228.794028)
  line L1590 (38.276389, 232.180694) -> (38.276389, 229.040972)
  line L1591 (38.593889, 232.498194) -> (38.452778, 232.498194)
  line L1592 (38.452778, 232.498194) -> (38.311667, 232.392361)
  line L1593 (37.923611, 223.114305) -> (37.7825, 223.149583)
  line L1594 (19.296944, 281.745972) -> (22.436667, 284.885694)